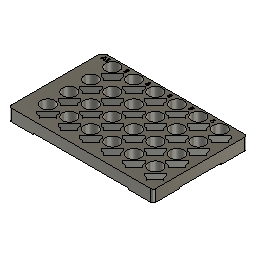
opentrons-tuberack-insert (Autodesk Fusion 360 design; units mm, degrees)
description: STEP AP214
part number: OpenTrons_1.5mL_rack
Autodesk Fusion 360 part; units mm, degrees
note: some values were not read from the file. Chosen so that the rebuilt part matches the saved one: which face or edge a step refers to.
(part 1 of 2)
imported_body "Base Feature1" makes body 1
other "Base Mesh Feature1"
sketch "Sketch1" plane through (0, 0, 0) normal (0, 0, 1) x (1, 0, 0)
  line L0 (-117.6969, -5.1718) -> (-116.414, -1.9968)
  line L1 (-116.414, -1.9968) -> (-115.8855, -1.9968)
  line L2 (-115.8855, -1.9968) -> (-114.6033, -5.1718)
  line L3 (-114.6033, -5.1718) -> (-115.2119, -5.1718)
  line L4 (-115.2119, -5.1718) -> (-115.4587, -4.5205)
  line L5 (-115.4587, -4.5205) -> (-116.8421, -4.5205)
  line L6 (-116.8421, -4.5205) -> (-117.0888, -5.1718)
  line L7 (-117.0888, -5.1718) -> (-117.6969, -5.1718)
  spline S0 degree 3 poles (-97.512, -2.4852) (-97.5271, -2.4858) (-97.5568, -2.4868) (-97.6004, -2.4938) (-97.6419, -2.5061) (-97.6818, -2.5226) (-97.7196, -2.5445) (-97.7552, -2.5715) (-97.789, -2.6028) (-97.8209, -2.6385) (-97.8499, -2.6783) (-97.8756, -2.7219) (-97.8969, -2.7692) (-97.9157, -2.8197) (-97.9302, -2.8738) (-97.9407, -2.9312) (-97.9487, -2.9919) (-97.9506, -3.0337) (-97.9515, -3.0551) knots 0 0 0 0 0.056467 0.111164 0.164937 0.218322 0.272393 0.327976 0.385291 0.444903 0.506844 0.569488 0.634153 0.700976 0.770897 0.843626 0.91966 1 1 1 1
  line L8 (-97.9515, -3.0551) -> (-98.5214, -3.0551)
  spline S1 degree 3 poles (-98.5214, -3.0551) (-98.5189, -3.012) (-98.5141, -2.9278) (-98.495, -2.8054) (-98.4693, -2.6898) (-98.4351, -2.5814) (-98.3922, -2.4801) (-98.3415, -2.3857) (-98.2819, -2.2986) (-98.2146, -2.2192) (-98.1407, -2.1481) (-98.0618, -2.085) (-97.9767, -2.0329) (-97.8869, -1.99) (-97.7924, -1.9558) (-97.6924, -1.9329) (-97.5878, -1.9174) (-97.5161, -1.9161) (-97.4796, -1.9154) knots 0 0 0 0 0.07494 0.146428 0.214753 0.280422 0.343604 0.405543 0.466199 0.526538 0.585902 0.64409 0.701613 0.758754 0.816629 0.875655 0.936624 1 1 1 1
  spline S2 degree 3 poles (-97.4796, -1.9154) (-97.4347, -1.9168) (-97.3472, -1.9195) (-97.22, -1.9428) (-97.1013, -1.9818) (-96.991, -2.0362) (-96.8902, -2.1054) (-96.7988, -2.1878) (-96.7196, -2.2854) (-96.6521, -2.3938) (-96.5961, -2.5087) (-96.5568, -2.6275) (-96.5309, -2.747) (-96.5282, -2.8275) (-96.5268, -2.8675) knots 0 0 0 0 0.089615 0.174949 0.257548 0.338901 0.420053 0.501401 0.584252 0.67037 0.756473 0.839207 0.92012 1 1 1 1
  spline S3 degree 3 poles (-96.5268, -2.8675) (-96.5274, -2.8917) (-96.5284, -2.9404) (-96.5359, -3.014) (-96.5471, -3.0891) (-96.5639, -3.1654) (-96.585, -3.2431) (-96.6105, -3.3223) (-96.6411, -3.4027) (-96.6762, -3.485) (-96.7181, -3.5697) (-96.767, -3.6579) (-96.824, -3.7495) (-96.8885, -3.8452) (-96.9608, -3.9447) (-97.0413, -4.0477) (-97.129, -4.1547) (-97.1913, -4.2262) (-97.2233, -4.2629) knots 0 0 0 0 0.045518 0.091616 0.139247 0.188242 0.238673 0.290664 0.34484 0.400432 0.459144 0.522551 0.590101 0.66226 0.739681 0.821575 0.90833 1 1 1 1
  line L9 (-97.2233, -4.2629) -> (-97.5546, -4.6426)
  line L10 (-97.5546, -4.6426) -> (-96.4861, -4.6426)
  line L11 (-96.4861, -4.6426) -> (-96.4861, -5.1718)
  line L12 (-96.4861, -5.1718) -> (-98.6028, -5.1718)
  line L13 (-98.6028, -5.1718) -> (-98.6028, -4.883)
  line L14 (-98.6028, -4.883) -> (-97.6628, -3.8826)
  spline S4 degree 3 poles (-97.6628, -3.8826) (-97.6355, -3.8534) (-97.5828, -3.7969) (-97.5078, -3.7139) (-97.44, -3.6351) (-97.3806, -3.5597) (-97.3267, -3.4902) (-97.2806, -3.4244) (-97.242, -3.363) (-97.2, -3.2889) (-97.1601, -3.2005) (-97.1236, -3.0987) (-97.1013, -3.0014) (-97.0982, -2.938) (-97.0967, -2.9076) knots 0 0 0 0 0.103844 0.201115 0.291116 0.374348 0.450707 0.52004 0.583258 0.639578 0.741537 0.83506 0.920873 1 1 1 1
  spline S5 degree 3 poles (-97.0967, -2.9076) (-97.0978, -2.8781) (-97.0999, -2.8211) (-97.1234, -2.74) (-97.1599, -2.6666) (-97.2112, -2.603) (-97.2734, -2.5508) (-97.3452, -2.5119) (-97.4261, -2.4895) (-97.4828, -2.4867) (-97.512, -2.4852) knots 0 0 0 0 0.132755 0.257234 0.378601 0.501406 0.623942 0.743642 0.868121 1 1 1 1
  line L15 (-62.7047, -3.9436) -> (-61.3856, -1.9154)
  line L16 (-61.3856, -1.9154) -> (-60.7916, -1.9154)
  line L17 (-60.7916, -1.9154) -> (-60.7916, -3.9913)
  line L18 (-60.7916, -3.9913) -> (-60.5066, -3.9913)
  line L19 (-60.5066, -3.9913) -> (-60.5066, -4.5205)
  line L20 (-60.5066, -4.5205) -> (-60.7916, -4.5205)
  line L21 (-60.7916, -4.5205) -> (-60.7916, -5.1718)
  line L22 (-60.7916, -5.1718) -> (-61.3614, -5.1718)
  line L23 (-61.3614, -5.1718) -> (-61.3614, -4.5205)
  line L24 (-61.3614, -4.5205) -> (-62.7047, -4.5205)
  line L25 (-62.7047, -4.5205) -> (-62.7047, -3.9436)
  line L26 (-25.9665, -3.5003) -> (-25.1601, -1.9154)
  line L27 (-25.1601, -1.9154) -> (-24.6557, -2.1711)
  line L28 (-24.6557, -2.1711) -> (-25.209, -3.2586)
  spline S6 degree 3 poles (-25.209, -3.2586) (-25.1763, -3.2595) (-25.112, -3.2612) (-25.0172, -3.2746) (-24.9266, -3.2979) (-24.8393, -3.3288) (-24.7563, -3.3703) (-24.6763, -3.4196) (-24.6014, -3.4797) (-24.5297, -3.5464) (-24.4646, -3.6202) (-24.408, -3.6996) (-24.3587, -3.7825) (-24.3204, -3.8708) (-24.2895, -3.9631) (-24.2672, -4.0598) (-24.2545, -4.161) (-24.2527, -4.2298) (-24.2518, -4.2648) knots 0 0 0 0 0.063329 0.124736 0.184916 0.2443 0.303826 0.364353 0.426073 0.489721 0.553756 0.616458 0.678319 0.740301 0.802656 0.866732 0.932157 1 1 1 1
  spline S7 degree 3 poles (-24.2518, -4.2648) (-24.2527, -4.2986) (-24.2543, -4.3653) (-24.268, -4.4633) (-24.2901, -4.5573) (-24.3217, -4.6471) (-24.3618, -4.7333) (-24.4109, -4.8156) (-24.4694, -4.8936) (-24.5357, -4.9668) (-24.6082, -5.0335) (-24.6846, -5.0927) (-24.7655, -5.1417) (-24.8495, -5.1831) (-24.9381, -5.2139) (-25.03, -5.2372) (-25.1257, -5.2506) (-25.1908, -5.2523) (-25.2237, -5.2532) knots 0 0 0 0 0.065621 0.129704 0.192008 0.253165 0.31459 0.376533 0.439287 0.503799 0.568284 0.630629 0.691513 0.751998 0.812377 0.873577 0.936027 1 1 1 1
  spline S8 degree 3 poles (-25.2237, -5.2532) (-25.2581, -5.2525) (-25.3257, -5.2511) (-25.4247, -5.2357) (-25.5197, -5.2124) (-25.61, -5.1792) (-25.6964, -5.1369) (-25.7776, -5.0845) (-25.8546, -5.0227) (-25.9264, -4.9529) (-25.991, -4.8763) (-26.0487, -4.7969) (-26.0975, -4.7143) (-26.137, -4.6289) (-26.1678, -4.5407) (-26.1892, -4.4496) (-26.2032, -4.356) (-26.2048, -4.2924) (-26.2057, -4.2604) knots 0 0 0 0 0.066486 0.130736 0.193287 0.255291 0.316538 0.378867 0.441877 0.507117 0.572271 0.635427 0.696817 0.757357 0.817265 0.877134 0.93802 1 1 1 1
  spline S9 degree 3 poles (-26.2057, -4.2604) (-26.2052, -4.2355) (-26.2044, -4.1857) (-26.1956, -4.1112) (-26.1822, -4.0364) (-26.1667, -3.9733) (-26.1507, -3.92) (-26.1346, -3.8748) (-26.1147, -3.8247) (-26.092, -3.7695) (-26.0656, -3.7093) (-26.0359, -3.6443) (-26.0026, -3.5739) (-25.9789, -3.5255) (-25.9665, -3.5003) knots 0 0 0 0 0.092538 0.185591 0.279552 0.375602 0.427617 0.487117 0.554199 0.628624 0.709688 0.799181 0.895357 1 1 1 1
  line L29 (-44.2093, -3.7586) -> (-43.836, -1.9968)
  line L30 (-43.836, -1.9968) -> (-42.3903, -1.9968)
  line L31 (-42.3903, -1.9968) -> (-42.3903, -2.5259)
  line L32 (-42.3903, -2.5259) -> (-43.3844, -2.5259)
  line L33 (-43.3844, -2.5259) -> (-43.5084, -3.1264)
  spline S10 degree 3 poles (-43.5084, -3.1264) (-43.4915, -3.1216) (-43.4582, -3.1124) (-43.408, -3.1031) (-43.3593, -3.097) (-43.3274, -3.0962) (-43.3119, -3.0958) knots 0 0 0 0 0.263654 0.51998 0.767103 1 1 1 1
  spline S11 degree 3 poles (-43.3119, -3.0958) (-43.2781, -3.0966) (-43.2116, -3.0981) (-43.1142, -3.1126) (-43.021, -3.1354) (-42.9322, -3.1679) (-42.8479, -3.2102) (-42.768, -3.2614) (-42.6924, -3.3216) (-42.6224, -3.3908) (-42.5582, -3.4667) (-42.5023, -3.5489) (-42.4546, -3.636) (-42.4166, -3.7288) (-42.3866, -3.8265) (-42.365, -3.9293) (-42.3522, -4.0372) (-42.3505, -4.1109) (-42.3496, -4.1484) knots 0 0 0 0 0.063401 0.124976 0.184492 0.243474 0.302264 0.361384 0.421482 0.483455 0.545936 0.608143 0.66982 0.732332 0.796092 0.861643 0.929435 1 1 1 1
  spline S12 degree 3 poles (-42.3496, -4.1484) (-42.3507, -4.1864) (-42.3528, -4.2614) (-42.3666, -4.3716) (-42.3911, -4.4771) (-42.4247, -4.5783) (-42.4689, -4.6744) (-42.5221, -4.7664) (-42.5852, -4.8535) (-42.6575, -4.935) (-42.7361, -5.0094) (-42.8199, -5.0749) (-42.9081, -5.13) (-43.0008, -5.1746) (-43.0975, -5.2098) (-43.1982, -5.2355) (-43.3034, -5.2502) (-43.3748, -5.2522) (-43.4111, -5.2532) knots 0 0 0 0 0.066755 0.131728 0.19481 0.256899 0.318751 0.380351 0.443324 0.507463 0.571506 0.633361 0.693942 0.753929 0.813802 0.874524 0.936222 1 1 1 1
  spline S13 degree 3 poles (-43.4111, -5.2532) (-43.4436, -5.2524) (-43.5076, -5.2507) (-43.6019, -5.2407) (-43.6928, -5.2229) (-43.7798, -5.1972) (-43.8639, -5.1655) (-43.9441, -5.1259) (-44.0208, -5.0791) (-44.0938, -5.0259) (-44.1619, -4.9661) (-44.224, -4.9006) (-44.2806, -4.8302) (-44.3304, -4.7542) (-44.3733, -4.6725) (-44.4113, -4.5862) (-44.4424, -4.4944) (-44.4582, -4.4307) (-44.4663, -4.3984) knots 0 0 0 0 0.065935 0.130037 0.192362 0.25382 0.314199 0.37467 0.435154 0.496479 0.557809 0.619031 0.679691 0.740961 0.803375 0.866818 0.932318 1 1 1 1
  line L34 (-44.4663, -4.3984) -> (-43.815, -4.3984)
  spline S14 degree 3 poles (-43.815, -4.3984) (-43.8031, -4.4208) (-43.7799, -4.4644) (-43.7359, -4.5222) (-43.6866, -4.5715) (-43.6326, -4.6128) (-43.5733, -4.6438) (-43.5113, -4.6672) (-43.4458, -4.6808) (-43.4012, -4.6825) (-43.3787, -4.6833) knots 0 0 0 0 0.138114 0.268408 0.394191 0.517092 0.637493 0.757004 0.877294 1 1 1 1
  spline S15 degree 3 poles (-43.3787, -4.6833) (-43.363, -4.6827) (-43.3321, -4.6816) (-43.2865, -4.6754) (-43.2431, -4.6638) (-43.2014, -4.6476) (-43.1613, -4.6275) (-43.1234, -4.6021) (-43.0871, -4.5729) (-43.0529, -4.5394) (-43.0219, -4.502) (-42.9947, -4.4618) (-42.9704, -4.4197) (-42.9524, -4.3741) (-42.9377, -4.3262) (-42.9268, -4.2758) (-42.9204, -4.2228) (-42.9198, -4.1866) (-42.9195, -4.1681) knots 0 0 0 0 0.061179 0.120371 0.178442 0.235934 0.294268 0.352654 0.413122 0.475586 0.5389 0.601869 0.664333 0.727647 0.792409 0.85912 0.928135 1 1 1 1
  spline S16 degree 3 poles (-42.9195, -4.1681) (-42.9198, -4.1501) (-42.9205, -4.115) (-42.9262, -4.0635) (-42.9365, -4.0146) (-42.9504, -3.9679) (-42.9683, -3.9238) (-42.9901, -3.882) (-43.016, -3.8427) (-43.0461, -3.8067) (-43.0782, -3.7736) (-43.1126, -3.7447) (-43.1492, -3.7207) (-43.1867, -3.6998) (-43.2266, -3.6846) (-43.268, -3.6741) (-43.311, -3.6664) (-43.3403, -3.6659) (-43.3551, -3.6657) knots 0 0 0 0 0.072891 0.141883 0.209282 0.274623 0.338439 0.401305 0.465006 0.52832 0.59074 0.650981 0.70969 0.767212 0.824188 0.881767 0.939955 1 1 1 1
  spline S17 degree 3 poles (-43.3551, -3.6657) (-43.3713, -3.6663) (-43.4037, -3.6675) (-43.4518, -3.6775) (-43.4993, -3.6937) (-43.5465, -3.716) (-43.593, -3.7453) (-43.6399, -3.7795) (-43.6856, -3.8213) (-43.7147, -3.8525) (-43.7297, -3.8686) knots 0 0 0 0 0.11036 0.221186 0.334364 0.452977 0.577234 0.708804 0.849355 1 1 1 1
  line L35 (-43.7297, -3.8686) -> (-44.2093, -3.7586)
  spline S18 degree 3 poles (-79.3483, -2.4852) (-79.369, -2.4863) (-79.41, -2.4883) (-79.4699, -2.5033) (-79.5268, -2.5287) (-79.5795, -2.5636) (-79.6272, -2.6056) (-79.6664, -2.6553) (-79.699, -2.7097) (-79.7128, -2.7499) (-79.7198, -2.7702) knots 0 0 0 0 0.123523 0.245107 0.367266 0.494691 0.622324 0.746003 0.872253 1 1 1 1
  line L36 (-79.7198, -2.7702) -> (-80.2896, -2.7702)
  spline S19 degree 3 poles (-80.2896, -2.7702) (-80.2856, -2.7417) (-80.2777, -2.6859) (-80.2589, -2.605) (-80.2363, -2.5283) (-80.2081, -2.456) (-80.175, -2.388) (-80.1375, -2.324) (-80.0949, -2.2644) (-80.0623, -2.2284) (-80.0461, -2.2105) knots 0 0 0 0 0.138934 0.272371 0.400702 0.524915 0.646775 0.765706 0.883115 1 1 1 1
  spline S20 degree 3 poles (-80.0461, -2.2105) (-80.0226, -2.1868) (-79.9764, -2.1402) (-79.8991, -2.0805) (-79.8181, -2.0288) (-79.7318, -1.9878) (-79.6414, -1.9546) (-79.5464, -1.9324) (-79.447, -1.9176) (-79.3791, -1.9161) (-79.3445, -1.9154) knots 0 0 0 0 0.127407 0.251106 0.372908 0.494496 0.616171 0.740563 0.867605 1 1 1 1
  spline S21 degree 3 poles (-79.3445, -1.9154) (-79.3138, -1.9161) (-79.2533, -1.9175) (-79.1644, -1.929) (-79.0796, -1.9491) (-78.9981, -1.9754) (-78.921, -2.0112) (-78.8467, -2.0527) (-78.7771, -2.1036) (-78.7123, -2.1612) (-78.6527, -2.2234) (-78.6011, -2.2899) (-78.5567, -2.359) (-78.5202, -2.4311) (-78.4921, -2.5064) (-78.4726, -2.5845) (-78.4598, -2.6652) (-78.4586, -2.7201) (-78.4579, -2.7479) knots 0 0 0 0 0.068214 0.134095 0.198286 0.26116 0.323635 0.386367 0.449642 0.514245 0.578413 0.640375 0.700615 0.760104 0.819299 0.878466 0.93836 1 1 1 1
  spline S22 degree 3 poles (-78.4579, -2.7479) (-78.4592, -2.7824) (-78.4618, -2.8502) (-78.4832, -2.9495) (-78.5167, -3.0444) (-78.565, -3.1337) (-78.6255, -3.217) (-78.6996, -3.2916) (-78.7854, -3.3587) (-78.8498, -3.3947) (-78.8828, -3.4132) knots 0 0 0 0 0.124101 0.244316 0.364466 0.485854 0.608915 0.734301 0.863943 1 1 1 1
  spline S23 degree 3 poles (-78.8828, -3.4132) (-78.8601, -3.4206) (-78.8157, -3.4352) (-78.7525, -3.464) (-78.6924, -3.4954) (-78.6364, -3.5319) (-78.584, -3.572) (-78.5355, -3.6161) (-78.4907, -3.664) (-78.4502, -3.716) (-78.4142, -3.7714) (-78.3819, -3.8287) (-78.3554, -3.8889) (-78.3329, -3.9513) (-78.3157, -4.0164) (-78.3037, -4.084) (-78.2967, -4.154) (-78.2956, -4.2014) (-78.2951, -4.2254) knots 0 0 0 0 0.066221 0.130122 0.192922 0.254764 0.315757 0.376303 0.436814 0.498168 0.559516 0.620243 0.68097 0.742349 0.804584 0.868102 0.933307 1 1 1 1
  spline S24 degree 3 poles (-78.2951, -4.2254) (-78.2962, -4.2606) (-78.2983, -4.3301) (-78.312, -4.4324) (-78.3374, -4.5299) (-78.3709, -4.6238) (-78.4155, -4.7129) (-78.4681, -4.7991) (-78.5326, -4.8796) (-78.6044, -4.9563) (-78.6841, -5.0261) (-78.7705, -5.0866) (-78.8617, -5.1385) (-78.9583, -5.1806) (-79.0602, -5.2131) (-79.1673, -5.2366) (-79.2799, -5.2509) (-79.3568, -5.2524) (-79.396, -5.2532) knots 0 0 0 0 0.062821 0.123871 0.183554 0.242266 0.301265 0.360847 0.421949 0.484789 0.548014 0.610413 0.672536 0.734829 0.797947 0.862973 0.93002 1 1 1 1
  spline S25 degree 3 poles (-79.396, -5.2532) (-79.4332, -5.2524) (-79.5058, -5.2508) (-79.6121, -5.2371) (-79.713, -5.215) (-79.809, -5.1838) (-79.8995, -5.1433) (-79.9856, -5.0952) (-80.0653, -5.0366) (-80.1396, -4.9701) (-80.2069, -4.8955) (-80.2671, -4.8145) (-80.3188, -4.7268) (-80.3622, -4.6329) (-80.397, -4.5324) (-80.4245, -4.4257) (-80.4436, -4.3125) (-80.4495, -4.2346) (-80.4525, -4.1949) knots 0 0 0 0 0.066659 0.130343 0.191936 0.251996 0.311122 0.369755 0.428602 0.488436 0.548524 0.608661 0.669236 0.730881 0.794196 0.85983 0.928533 1 1 1 1
  line L37 (-80.4525, -4.1949) -> (-79.8826, -4.1949)
  spline S26 degree 3 poles (-79.8826, -4.1949) (-79.879, -4.2148) (-79.872, -4.2537) (-79.8582, -4.31) (-79.8404, -4.362) (-79.8197, -4.4101) (-79.7974, -4.455) (-79.7704, -4.495) (-79.7407, -4.5311) (-79.6979, -4.5741) (-79.6368, -4.6183) (-79.5542, -4.6567) (-79.4623, -4.6792) (-79.3981, -4.6819) (-79.3649, -4.6833) knots 0 0 0 0 0.077346 0.150652 0.220677 0.286575 0.350188 0.411379 0.469946 0.528234 0.642194 0.755364 0.873556 1 1 1 1
  spline S27 degree 3 poles (-79.3649, -4.6833) (-79.3473, -4.683) (-79.3128, -4.6824) (-79.2621, -4.6759) (-79.2138, -4.6651) (-79.1678, -4.6504) (-79.1239, -4.632) (-79.0828, -4.6083) (-79.0437, -4.5807) (-79.007, -4.5497) (-78.9732, -4.5159) (-78.945, -4.4784) (-78.9193, -4.4404) (-78.9002, -4.3993) (-78.8836, -4.3573) (-78.8734, -4.3129) (-78.8656, -4.267) (-78.8652, -4.2356) (-78.865, -4.2197) knots 0 0 0 0 0.069402 0.135943 0.20102 0.264181 0.325955 0.388454 0.450819 0.514266 0.577492 0.638835 0.698634 0.758057 0.817032 0.876415 0.937278 1 1 1 1
  spline S28 degree 3 poles (-78.865, -4.2197) (-78.8656, -4.2022) (-78.8668, -4.1675) (-78.8766, -4.1169) (-78.8921, -4.0682) (-78.9136, -4.0216) (-78.9424, -3.9774) (-78.9763, -3.9346) (-79.0181, -3.8954) (-79.064, -3.8567) (-79.1172, -3.823) (-79.1751, -3.7918) (-79.2392, -3.7671) (-79.308, -3.7449) (-79.3829, -3.7288) (-79.4632, -3.717) (-79.5489, -3.7083) (-79.608, -3.707) (-79.6384, -3.7064) knots 0 0 0 0 0.050613 0.10076 0.149275 0.198888 0.249306 0.302323 0.357221 0.415437 0.476443 0.539829 0.606184 0.675941 0.749782 0.828288 0.911845 1 1 1 1
  line L38 (-79.6384, -3.7064) -> (-79.6384, -3.1772)
  spline S29 degree 3 poles (-79.6384, -3.1772) (-79.6006, -3.174) (-79.5299, -3.168) (-79.4318, -3.1539) (-79.3492, -3.1351) (-79.2802, -3.1124) (-79.2229, -3.0833) (-79.1728, -3.0511) (-79.1296, -3.0137) (-79.0932, -2.9723) (-79.064, -2.9278) (-79.0434, -2.8809) (-79.0297, -2.8331) (-79.0284, -2.8004) (-79.0278, -2.7842) knots 0 0 0 0 0.141704 0.2651 0.370058 0.458024 0.535994 0.609848 0.680075 0.748587 0.81563 0.878071 0.939584 1 1 1 1
  spline S30 degree 3 poles (-79.0278, -2.7842) (-79.0289, -2.7635) (-79.031, -2.7232) (-79.0478, -2.6654) (-79.0768, -2.6139) (-79.1158, -2.5688) (-79.1633, -2.5312) (-79.2189, -2.5038) (-79.2815, -2.4878) (-79.3256, -2.4861) (-79.3483, -2.4852) knots 0 0 0 0 0.126208 0.246331 0.363484 0.484754 0.608383 0.731214 0.860989 1 1 1 1
  line L39 (-114.1352, -2.5259) -> (-113.7949, -1.9968)
  line L40 (-113.7949, -1.9968) -> (-112.914, -1.9968)
  line L41 (-112.914, -1.9968) -> (-112.914, -5.1718)
  line L42 (-112.914, -5.1718) -> (-113.4839, -5.1718)
  line L43 (-113.4839, -5.1718) -> (-113.4839, -2.5259)
  line L44 (-113.4839, -2.5259) -> (-114.1352, -2.5259)
  line L45 (-2, 0) -> (-117, 0)
  line L46 (-121, -4) -> (-121, -76.75)
  line L47 (-119, -78.75) -> (-2, -78.75)
  line L48 (0, -76.75) -> (0, -2)
  line L49 (-16.0663, -16.324) -> (-6.591, -6.8487)
  line L50 (-4.8233, -8.6165) -> (-6.591, -6.8487)
  line L51 (-4.8233, -8.6165) -> (-4.2576, -11.5864)
  line L52 (-4.2576, -11.5864) -> (-11.3286, -18.6574)
  line L53 (-11.3286, -18.6574) -> (-14.2985, -18.0917)
  line L54 (-14.2985, -18.0917) -> (-16.0663, -16.324)
  line L55 (-11.3286, -11.5864) -> (-16.19, -6.725) construction
  line L56 (-121, -4) -> (-117, 0)
  circle A0 centre (-16.19, -6.725) radius 5.675
  arc A1 (0, -2) -> (-2, 0) centre (-2, -2) ccw
  arc A2 (-2, -78.75) -> (0, -76.75) centre (-2, -76.75) ccw
  arc A3 (-121, -76.75) -> (-119, -78.75) centre (-119, -76.75) ccw
  line L57 (-100.5, -78.75) -> (-100.5, -76.75)
  line L58 (-20.5, -76.75) -> (-20.5, -78.75)
  line L59 (-20.5, -76.75) -> (-100.5, -76.75)
  line L60 (0, -39.375) -> (-121, -39.375) construction
  line L61 (-20.5, -2) -> (-100.5, -2)
  line L62 (-100.5, 0) -> (-100.5, -2)
  line L63 (-20.5, -2) -> (-20.5, 0)
  line L64 (-11.3286, -18.6574) -> (-9.9144, -20.0716)
  line L65 (-9.9144, -20.0716) -> (-2.8434, -13.0006)
  line L66 (-2.8434, -13.0006) -> (-4.2576, -11.5864)
  line L67 (-16.19, -6.725) -> (0, -6.725) construction
  line L68 (-98.5214, -3.0551) -> (-98.5189, -3.012) construction
  line L69 (-98.5189, -3.012) -> (-98.5141, -2.9278) construction
  line L70 (-98.5141, -2.9278) -> (-98.495, -2.8054) construction
  line L71 (-98.495, -2.8054) -> (-98.4693, -2.6898) construction
  line L72 (-98.4693, -2.6898) -> (-98.4351, -2.5814) construction
  line L73 (-98.4351, -2.5814) -> (-98.3922, -2.4801) construction
  line L74 (-98.3922, -2.4801) -> (-98.3415, -2.3857) construction
  line L75 (-98.3415, -2.3857) -> (-98.2819, -2.2986) construction
  line L76 (-98.2819, -2.2986) -> (-98.2146, -2.2192) construction
  line L77 (-98.2146, -2.2192) -> (-98.1407, -2.1481) construction
  line L78 (-98.1407, -2.1481) -> (-98.0618, -2.085) construction
  line L79 (-98.0618, -2.085) -> (-97.9767, -2.0329) construction
  line L80 (-97.9767, -2.0329) -> (-97.8869, -1.99) construction
  line L81 (-97.8869, -1.99) -> (-97.7924, -1.9558) construction
  line L82 (-97.7924, -1.9558) -> (-97.6924, -1.9329) construction
  line L83 (-97.6924, -1.9329) -> (-97.5878, -1.9174) construction
  line L84 (-97.5878, -1.9174) -> (-97.5161, -1.9161) construction
  line L85 (-97.5161, -1.9161) -> (-97.4796, -1.9154) construction
  line L86 (-97.4796, -1.9154) -> (-97.4347, -1.9168) construction
  line L87 (-97.4347, -1.9168) -> (-97.3472, -1.9195) construction
  line L88 (-97.3472, -1.9195) -> (-97.22, -1.9428) construction
  line L89 (-97.22, -1.9428) -> (-97.1013, -1.9818) construction
  line L90 (-97.1013, -1.9818) -> (-96.991, -2.0362) construction
  line L91 (-96.991, -2.0362) -> (-96.8902, -2.1054) construction
  line L92 (-96.8902, -2.1054) -> (-96.7988, -2.1878) construction
  line L93 (-96.7988, -2.1878) -> (-96.7196, -2.2854) construction
  line L94 (-96.7196, -2.2854) -> (-96.6521, -2.3938) construction
  line L95 (-96.6521, -2.3938) -> (-96.5961, -2.5087) construction
  line L96 (-96.5961, -2.5087) -> (-96.5568, -2.6275) construction
  line L97 (-96.5568, -2.6275) -> (-96.5309, -2.747) construction
  line L98 (-96.5309, -2.747) -> (-96.5282, -2.8275) construction
  line L99 (-96.5282, -2.8275) -> (-96.5268, -2.8675) construction
  line L100 (-97.6628, -3.8826) -> (-97.6355, -3.8534) construction
  line L101 (-97.6355, -3.8534) -> (-97.5828, -3.7969) construction
  line L102 (-97.5828, -3.7969) -> (-97.5078, -3.7139) construction
  line L103 (-97.5078, -3.7139) -> (-97.44, -3.6351) construction
  line L104 (-97.44, -3.6351) -> (-97.3806, -3.5597) construction
  line L105 (-97.3806, -3.5597) -> (-97.3267, -3.4902) construction
  line L106 (-97.3267, -3.4902) -> (-97.2806, -3.4244) construction
  line L107 (-97.2806, -3.4244) -> (-97.242, -3.363) construction
  line L108 (-97.242, -3.363) -> (-97.2, -3.2889) construction
  line L109 (-97.2, -3.2889) -> (-97.1601, -3.2005) construction
  line L110 (-97.1601, -3.2005) -> (-97.1236, -3.0987) construction
  line L111 (-97.1236, -3.0987) -> (-97.1013, -3.0014) construction
  line L112 (-97.1013, -3.0014) -> (-97.0982, -2.938) construction
  line L113 (-97.0982, -2.938) -> (-97.0967, -2.9076) construction
  line L114 (-97.512, -2.4852) -> (-97.5271, -2.4858) construction
  line L115 (-97.5271, -2.4858) -> (-97.5568, -2.4868) construction
  line L116 (-97.5568, -2.4868) -> (-97.6004, -2.4938) construction
  line L117 (-97.6004, -2.4938) -> (-97.6419, -2.5061) construction
  line L118 (-97.6419, -2.5061) -> (-97.6818, -2.5226) construction
  line L119 (-97.6818, -2.5226) -> (-97.7196, -2.5445) construction
  line L120 (-97.7196, -2.5445) -> (-97.7552, -2.5715) construction
  line L121 (-97.7552, -2.5715) -> (-97.789, -2.6028) construction
  line L122 (-97.789, -2.6028) -> (-97.8209, -2.6385) construction
  line L123 (-97.8209, -2.6385) -> (-97.8499, -2.6783) construction
  line L124 (-97.8499, -2.6783) -> (-97.8756, -2.7219) construction
  line L125 (-97.8756, -2.7219) -> (-97.8969, -2.7692) construction
  line L126 (-97.8969, -2.7692) -> (-97.9157, -2.8197) construction
  line L127 (-97.9157, -2.8197) -> (-97.9302, -2.8738) construction
  line L128 (-97.9302, -2.8738) -> (-97.9407, -2.9312) construction
  line L129 (-97.9407, -2.9312) -> (-97.9487, -2.9919) construction
  line L130 (-97.9487, -2.9919) -> (-97.9506, -3.0337) construction
  line L131 (-97.9506, -3.0337) -> (-97.9515, -3.0551) construction
  line L132 (-97.0967, -2.9076) -> (-97.0978, -2.8781) construction
  line L133 (-97.0978, -2.8781) -> (-97.0999, -2.8211) construction
  line L134 (-97.0999, -2.8211) -> (-97.1234, -2.74) construction
  line L135 (-97.1234, -2.74) -> (-97.1599, -2.6666) construction
  line L136 (-97.1599, -2.6666) -> (-97.2112, -2.603) construction
  line L137 (-97.2112, -2.603) -> (-97.2734, -2.5508) construction
  line L138 (-97.2734, -2.5508) -> (-97.3452, -2.5119) construction
  line L139 (-97.3452, -2.5119) -> (-97.4261, -2.4895) construction
  line L140 (-97.4261, -2.4895) -> (-97.4828, -2.4867) construction
  line L141 (-97.4828, -2.4867) -> (-97.512, -2.4852) construction
  line L142 (-96.5268, -2.8675) -> (-96.5274, -2.8917) construction
  line L143 (-96.5274, -2.8917) -> (-96.5284, -2.9404) construction
  line L144 (-96.5284, -2.9404) -> (-96.5359, -3.014) construction
  line L145 (-96.5359, -3.014) -> (-96.5471, -3.0891) construction
  line L146 (-96.5471, -3.0891) -> (-96.5639, -3.1654) construction
  line L147 (-96.5639, -3.1654) -> (-96.585, -3.2431) construction
  line L148 (-96.585, -3.2431) -> (-96.6105, -3.3223) construction
  line L149 (-96.6105, -3.3223) -> (-96.6411, -3.4027) construction
  line L150 (-96.6411, -3.4027) -> (-96.6762, -3.485) construction
  line L151 (-96.6762, -3.485) -> (-96.7181, -3.5697) construction
  line L152 (-96.7181, -3.5697) -> (-96.767, -3.6579) construction
  line L153 (-96.767, -3.6579) -> (-96.824, -3.7495) construction
  line L154 (-96.824, -3.7495) -> (-96.8885, -3.8452) construction
  line L155 (-96.8885, -3.8452) -> (-96.9608, -3.9447) construction
  line L156 (-96.9608, -3.9447) -> (-97.0413, -4.0477) construction
  line L157 (-97.0413, -4.0477) -> (-97.129, -4.1547) construction
  line L158 (-97.129, -4.1547) -> (-97.1913, -4.2262) construction
  line L159 (-97.1913, -4.2262) -> (-97.2233, -4.2629) construction
  line L160 (-79.396, -5.2532) -> (-79.4332, -5.2524) construction
  line L161 (-79.4332, -5.2524) -> (-79.5058, -5.2508) construction
  line L162 (-79.5058, -5.2508) -> (-79.6121, -5.2371) construction
  line L163 (-79.6121, -5.2371) -> (-79.713, -5.215) construction
  line L164 (-79.713, -5.215) -> (-79.809, -5.1838) construction
  line L165 (-79.809, -5.1838) -> (-79.8995, -5.1433) construction
  line L166 (-79.8995, -5.1433) -> (-79.9856, -5.0952) construction
  line L167 (-79.9856, -5.0952) -> (-80.0653, -5.0366) construction
  line L168 (-80.0653, -5.0366) -> (-80.1396, -4.9701) construction
  line L169 (-80.1396, -4.9701) -> (-80.2069, -4.8955) construction
  line L170 (-80.2069, -4.8955) -> (-80.2671, -4.8145) construction
  line L171 (-80.2671, -4.8145) -> (-80.3188, -4.7268) construction
  line L172 (-80.3188, -4.7268) -> (-80.3622, -4.6329) construction
  line L173 (-80.3622, -4.6329) -> (-80.397, -4.5324) construction
  line L174 (-80.397, -4.5324) -> (-80.4245, -4.4257) construction
  line L175 (-80.4245, -4.4257) -> (-80.4436, -4.3125) construction
  line L176 (-80.4436, -4.3125) -> (-80.4495, -4.2346) construction
  line L177 (-80.4495, -4.2346) -> (-80.4525, -4.1949) construction
  line L178 (-79.8826, -4.1949) -> (-79.879, -4.2148) construction
  line L179 (-79.879, -4.2148) -> (-79.872, -4.2537) construction
  line L180 (-79.872, -4.2537) -> (-79.8582, -4.31) construction
  line L181 (-79.8582, -4.31) -> (-79.8404, -4.362) construction
  line L182 (-79.8404, -4.362) -> (-79.8197, -4.4101) construction
  line L183 (-79.8197, -4.4101) -> (-79.7974, -4.455) construction
  line L184 (-79.7974, -4.455) -> (-79.7704, -4.495) construction
  line L185 (-79.7704, -4.495) -> (-79.7407, -4.5311) construction
  line L186 (-79.7407, -4.5311) -> (-79.6979, -4.5741) construction
  line L187 (-79.6979, -4.5741) -> (-79.6368, -4.6183) construction
  line L188 (-79.6368, -4.6183) -> (-79.5542, -4.6567) construction
  line L189 (-79.5542, -4.6567) -> (-79.4623, -4.6792) construction
  line L190 (-79.4623, -4.6792) -> (-79.3981, -4.6819) construction
  line L191 (-79.3981, -4.6819) -> (-79.3649, -4.6833) construction
  line L192 (-79.3649, -4.6833) -> (-79.3473, -4.683) construction
  line L193 (-79.3473, -4.683) -> (-79.3128, -4.6824) construction
  line L194 (-79.3128, -4.6824) -> (-79.2621, -4.6759) construction
  line L195 (-79.2621, -4.6759) -> (-79.2138, -4.6651) construction
  line L196 (-79.2138, -4.6651) -> (-79.1678, -4.6504) construction
  line L197 (-79.1678, -4.6504) -> (-79.1239, -4.632) construction
  line L198 (-79.1239, -4.632) -> (-79.0828, -4.6083) construction
  line L199 (-79.0828, -4.6083) -> (-79.0437, -4.5807) construction
  line L200 (-79.0437, -4.5807) -> (-79.007, -4.5497) construction
  line L201 (-79.007, -4.5497) -> (-78.9732, -4.5159) construction
  line L202 (-78.9732, -4.5159) -> (-78.945, -4.4784) construction
  line L203 (-78.945, -4.4784) -> (-78.9193, -4.4404) construction
  line L204 (-78.9193, -4.4404) -> (-78.9002, -4.3993) construction
  line L205 (-78.9002, -4.3993) -> (-78.8836, -4.3573) construction
  line L206 (-78.8836, -4.3573) -> (-78.8734, -4.3129) construction
  line L207 (-78.8734, -4.3129) -> (-78.8656, -4.267) construction
  line L208 (-78.8656, -4.267) -> (-78.8652, -4.2356) construction
  line L209 (-78.8652, -4.2356) -> (-78.865, -4.2197) construction
  line L210 (-78.865, -4.2197) -> (-78.8656, -4.2022) construction
  line L211 (-78.8656, -4.2022) -> (-78.8668, -4.1675) construction
  line L212 (-78.8668, -4.1675) -> (-78.8766, -4.1169) construction
  line L213 (-78.8766, -4.1169) -> (-78.8921, -4.0682) construction
  line L214 (-78.8921, -4.0682) -> (-78.9136, -4.0216) construction
  line L215 (-78.9136, -4.0216) -> (-78.9424, -3.9774) construction
  line L216 (-78.9424, -3.9774) -> (-78.9763, -3.9346) construction
  line L217 (-78.9763, -3.9346) -> (-79.0181, -3.8954) construction
  line L218 (-79.0181, -3.8954) -> (-79.064, -3.8567) construction
  line L219 (-79.064, -3.8567) -> (-79.1172, -3.823) construction
  line L220 (-79.1172, -3.823) -> (-79.1751, -3.7918) construction
  line L221 (-79.1751, -3.7918) -> (-79.2392, -3.7671) construction
  line L222 (-79.2392, -3.7671) -> (-79.308, -3.7449) construction
  line L223 (-79.308, -3.7449) -> (-79.3829, -3.7288) construction
  line L224 (-79.3829, -3.7288) -> (-79.4632, -3.717) construction
  line L225 (-79.4632, -3.717) -> (-79.5489, -3.7083) construction
  line L226 (-79.5489, -3.7083) -> (-79.608, -3.707) construction
  line L227 (-79.608, -3.707) -> (-79.6384, -3.7064) construction
  line L228 (-79.6384, -3.1772) -> (-79.6006, -3.174) construction
  line L229 (-79.6006, -3.174) -> (-79.5299, -3.168) construction
  line L230 (-79.5299, -3.168) -> (-79.4318, -3.1539) construction
  line L231 (-79.4318, -3.1539) -> (-79.3492, -3.1351) construction
  line L232 (-79.3492, -3.1351) -> (-79.2802, -3.1124) construction
  line L233 (-79.2802, -3.1124) -> (-79.2229, -3.0833) construction
  line L234 (-79.2229, -3.0833) -> (-79.1728, -3.0511) construction
  line L235 (-79.1728, -3.0511) -> (-79.1296, -3.0137) construction
  line L236 (-79.1296, -3.0137) -> (-79.0932, -2.9723) construction
  line L237 (-79.0932, -2.9723) -> (-79.064, -2.9278) construction
  line L238 (-79.064, -2.9278) -> (-79.0434, -2.8809) construction
  line L239 (-79.0434, -2.8809) -> (-79.0297, -2.8331) construction
  line L240 (-79.0297, -2.8331) -> (-79.0284, -2.8004) construction
  line L241 (-79.0284, -2.8004) -> (-79.0278, -2.7842) construction
  line L242 (-79.0278, -2.7842) -> (-79.0289, -2.7635) construction
  line L243 (-79.0289, -2.7635) -> (-79.031, -2.7232) construction
  line L244 (-79.031, -2.7232) -> (-79.0478, -2.6654) construction
  line L245 (-79.0478, -2.6654) -> (-79.0768, -2.6139) construction
  line L246 (-79.0768, -2.6139) -> (-79.1158, -2.5688) construction
  line L247 (-79.1158, -2.5688) -> (-79.1633, -2.5312) construction
  line L248 (-79.1633, -2.5312) -> (-79.2189, -2.5038) construction
  line L249 (-79.2189, -2.5038) -> (-79.2815, -2.4878) construction
  line L250 (-79.2815, -2.4878) -> (-79.3256, -2.4861) construction
  line L251 (-79.3256, -2.4861) -> (-79.3483, -2.4852) construction
  line L252 (-79.3483, -2.4852) -> (-79.369, -2.4863) construction
  line L253 (-79.369, -2.4863) -> (-79.41, -2.4883) construction
  line L254 (-79.41, -2.4883) -> (-79.4699, -2.5033) construction
  line L255 (-79.4699, -2.5033) -> (-79.5268, -2.5287) construction
  line L256 (-79.5268, -2.5287) -> (-79.5795, -2.5636) construction
  line L257 (-79.5795, -2.5636) -> (-79.6272, -2.6056) construction
  line L258 (-79.6272, -2.6056) -> (-79.6664, -2.6553) construction
  line L259 (-79.6664, -2.6553) -> (-79.699, -2.7097) construction
  line L260 (-79.699, -2.7097) -> (-79.7128, -2.7499) construction
  line L261 (-79.7128, -2.7499) -> (-79.7198, -2.7702) construction
  line L262 (-80.2896, -2.7702) -> (-80.2856, -2.7417) construction
  line L263 (-80.2856, -2.7417) -> (-80.2777, -2.6859) construction
  line L264 (-80.2777, -2.6859) -> (-80.2589, -2.605) construction
  line L265 (-80.2589, -2.605) -> (-80.2363, -2.5283) construction
  line L266 (-80.2363, -2.5283) -> (-80.2081, -2.456) construction
  line L267 (-80.2081, -2.456) -> (-80.175, -2.388) construction
  line L268 (-80.175, -2.388) -> (-80.1375, -2.324) construction
  line L269 (-80.1375, -2.324) -> (-80.0949, -2.2644) construction
  line L270 (-80.0949, -2.2644) -> (-80.0623, -2.2284) construction
  line L271 (-80.0623, -2.2284) -> (-80.0461, -2.2105) construction
  line L272 (-80.0461, -2.2105) -> (-80.0226, -2.1868) construction
  line L273 (-80.0226, -2.1868) -> (-79.9764, -2.1402) construction
  line L274 (-79.9764, -2.1402) -> (-79.8991, -2.0805) construction
  line L275 (-79.8991, -2.0805) -> (-79.8181, -2.0288) construction
  line L276 (-79.8181, -2.0288) -> (-79.7318, -1.9878) construction
  line L277 (-79.7318, -1.9878) -> (-79.6414, -1.9546) construction
  line L278 (-79.6414, -1.9546) -> (-79.5464, -1.9324) construction
  line L279 (-79.5464, -1.9324) -> (-79.447, -1.9176) construction
  line L280 (-79.447, -1.9176) -> (-79.3791, -1.9161) construction
  line L281 (-79.3791, -1.9161) -> (-79.3445, -1.9154) construction
  line L282 (-79.3445, -1.9154) -> (-79.3138, -1.9161) construction
  line L283 (-79.3138, -1.9161) -> (-79.2533, -1.9175) construction
  line L284 (-79.2533, -1.9175) -> (-79.1644, -1.929) construction
  line L285 (-79.1644, -1.929) -> (-79.0796, -1.9491) construction
  line L286 (-79.0796, -1.9491) -> (-78.9981, -1.9754) construction
  line L287 (-78.9981, -1.9754) -> (-78.921, -2.0112) construction
  line L288 (-78.921, -2.0112) -> (-78.8467, -2.0527) construction
  line L289 (-78.8467, -2.0527) -> (-78.7771, -2.1036) construction
  line L290 (-78.7771, -2.1036) -> (-78.7123, -2.1612) construction
  line L291 (-78.7123, -2.1612) -> (-78.6527, -2.2234) construction
  line L292 (-78.6527, -2.2234) -> (-78.6011, -2.2899) construction
  line L293 (-78.6011, -2.2899) -> (-78.5567, -2.359) construction
  line L294 (-78.5567, -2.359) -> (-78.5202, -2.4311) construction
  line L295 (-78.5202, -2.4311) -> (-78.4921, -2.5064) construction
  line L296 (-78.4921, -2.5064) -> (-78.4726, -2.5845) construction
  line L297 (-78.4726, -2.5845) -> (-78.4598, -2.6652) construction
  line L298 (-78.4598, -2.6652) -> (-78.4586, -2.7201) construction
  line L299 (-78.4586, -2.7201) -> (-78.4579, -2.7479) construction
  line L300 (-78.4579, -2.7479) -> (-78.4592, -2.7824) construction
  line L301 (-78.4592, -2.7824) -> (-78.4618, -2.8502) construction
  line L302 (-78.4618, -2.8502) -> (-78.4832, -2.9495) construction
  line L303 (-78.4832, -2.9495) -> (-78.5167, -3.0444) construction
  line L304 (-78.5167, -3.0444) -> (-78.565, -3.1337) construction
  line L305 (-78.565, -3.1337) -> (-78.6255, -3.217) construction
  line L306 (-78.6255, -3.217) -> (-78.6996, -3.2916) construction
  line L307 (-78.6996, -3.2916) -> (-78.7854, -3.3587) construction
  line L308 (-78.7854, -3.3587) -> (-78.8498, -3.3947) construction
  line L309 (-78.8498, -3.3947) -> (-78.8828, -3.4132) construction
  line L310 (-78.8828, -3.4132) -> (-78.8601, -3.4206) construction
  line L311 (-78.8601, -3.4206) -> (-78.8157, -3.4352) construction
  line L312 (-78.8157, -3.4352) -> (-78.7525, -3.464) construction
  line L313 (-78.7525, -3.464) -> (-78.6924, -3.4954) construction
  line L314 (-78.6924, -3.4954) -> (-78.6364, -3.5319) construction
  line L315 (-78.6364, -3.5319) -> (-78.584, -3.572) construction
  line L316 (-78.584, -3.572) -> (-78.5355, -3.6161) construction
  line L317 (-78.5355, -3.6161) -> (-78.4907, -3.664) construction
  line L318 (-78.4907, -3.664) -> (-78.4502, -3.716) construction
  line L319 (-78.4502, -3.716) -> (-78.4142, -3.7714) construction
  line L320 (-78.4142, -3.7714) -> (-78.3819, -3.8287) construction
  line L321 (-78.3819, -3.8287) -> (-78.3554, -3.8889) construction
  line L322 (-78.3554, -3.8889) -> (-78.3329, -3.9513) construction
  line L323 (-78.3329, -3.9513) -> (-78.3157, -4.0164) construction
  line L324 (-78.3157, -4.0164) -> (-78.3037, -4.084) construction
  line L325 (-78.3037, -4.084) -> (-78.2967, -4.154) construction
  line L326 (-78.2967, -4.154) -> (-78.2956, -4.2014) construction
  line L327 (-78.2956, -4.2014) -> (-78.2951, -4.2254) construction
  line L328 (-78.2951, -4.2254) -> (-78.2962, -4.2606) construction
  line L329 (-78.2962, -4.2606) -> (-78.2983, -4.3301) construction
  line L330 (-78.2983, -4.3301) -> (-78.312, -4.4324) construction
  line L331 (-78.312, -4.4324) -> (-78.3374, -4.5299) construction
  line L332 (-78.3374, -4.5299) -> (-78.3709, -4.6238) construction
  line L333 (-78.3709, -4.6238) -> (-78.4155, -4.7129) construction
  line L334 (-78.4155, -4.7129) -> (-78.4681, -4.7991) construction
  line L335 (-78.4681, -4.7991) -> (-78.5326, -4.8796) construction
  line L336 (-78.5326, -4.8796) -> (-78.6044, -4.9563) construction
  line L337 (-78.6044, -4.9563) -> (-78.6841, -5.0261) construction
  line L338 (-78.6841, -5.0261) -> (-78.7705, -5.0866) construction
  line L339 (-78.7705, -5.0866) -> (-78.8617, -5.1385) construction
  line L340 (-78.8617, -5.1385) -> (-78.9583, -5.1806) construction
  line L341 (-78.9583, -5.1806) -> (-79.0602, -5.2131) construction
  line L342 (-79.0602, -5.2131) -> (-79.1673, -5.2366) construction
  line L343 (-79.1673, -5.2366) -> (-79.2799, -5.2509) construction
  line L344 (-79.2799, -5.2509) -> (-79.3568, -5.2524) construction
  line L345 (-79.3568, -5.2524) -> (-79.396, -5.2532) construction
  line L346 (-43.5084, -3.1264) -> (-43.4915, -3.1216) construction
  line L347 (-43.4915, -3.1216) -> (-43.4582, -3.1124) construction
  line L348 (-43.4582, -3.1124) -> (-43.408, -3.1031) construction
  line L349 (-43.408, -3.1031) -> (-43.3593, -3.097) construction
  line L350 (-43.3593, -3.097) -> (-43.3274, -3.0962) construction
  line L351 (-43.3274, -3.0962) -> (-43.3119, -3.0958) construction
  line L352 (-43.3119, -3.0958) -> (-43.2781, -3.0966) construction
  line L353 (-43.2781, -3.0966) -> (-43.2116, -3.0981) construction
  line L354 (-43.2116, -3.0981) -> (-43.1142, -3.1126) construction
  line L355 (-43.1142, -3.1126) -> (-43.021, -3.1354) construction
  line L356 (-43.021, -3.1354) -> (-42.9322, -3.1679) construction
  line L357 (-42.9322, -3.1679) -> (-42.8479, -3.2102) construction
  line L358 (-42.8479, -3.2102) -> (-42.768, -3.2614) construction
  line L359 (-42.768, -3.2614) -> (-42.6924, -3.3216) construction
  line L360 (-42.6924, -3.3216) -> (-42.6224, -3.3908) construction
  line L361 (-42.6224, -3.3908) -> (-42.5582, -3.4667) construction
  line L362 (-42.5582, -3.4667) -> (-42.5023, -3.5489) construction
  line L363 (-42.5023, -3.5489) -> (-42.4546, -3.636) construction
  line L364 (-42.4546, -3.636) -> (-42.4166, -3.7288) construction
  line L365 (-42.4166, -3.7288) -> (-42.3866, -3.8265) construction
  line L366 (-42.3866, -3.8265) -> (-42.365, -3.9293) construction
  line L367 (-42.365, -3.9293) -> (-42.3522, -4.0372) construction
  line L368 (-42.3522, -4.0372) -> (-42.3505, -4.1109) construction
  line L369 (-42.3505, -4.1109) -> (-42.3496, -4.1484) construction
  line L370 (-42.3496, -4.1484) -> (-42.3507, -4.1864) construction
  line L371 (-42.3507, -4.1864) -> (-42.3528, -4.2614) construction
  line L372 (-42.3528, -4.2614) -> (-42.3666, -4.3716) construction
  line L373 (-42.3666, -4.3716) -> (-42.3911, -4.4771) construction
  line L374 (-42.3911, -4.4771) -> (-42.4247, -4.5783) construction
  line L375 (-42.4247, -4.5783) -> (-42.4689, -4.6744) construction
  line L376 (-42.4689, -4.6744) -> (-42.5221, -4.7664) construction
  line L377 (-42.5221, -4.7664) -> (-42.5852, -4.8535) construction
  line L378 (-42.5852, -4.8535) -> (-42.6575, -4.935) construction
  line L379 (-42.6575, -4.935) -> (-42.7361, -5.0094) construction
  line L380 (-42.7361, -5.0094) -> (-42.8199, -5.0749) construction
  line L381 (-42.8199, -5.0749) -> (-42.9081, -5.13) construction
  line L382 (-42.9081, -5.13) -> (-43.0008, -5.1746) construction
  line L383 (-43.0008, -5.1746) -> (-43.0975, -5.2098) construction
  line L384 (-43.0975, -5.2098) -> (-43.1982, -5.2355) construction
  line L385 (-43.1982, -5.2355) -> (-43.3034, -5.2502) construction
  line L386 (-43.3034, -5.2502) -> (-43.3748, -5.2522) construction
  line L387 (-43.3748, -5.2522) -> (-43.4111, -5.2532) construction
  line L388 (-43.4111, -5.2532) -> (-43.4436, -5.2524) construction
  line L389 (-43.4436, -5.2524) -> (-43.5076, -5.2507) construction
  line L390 (-43.5076, -5.2507) -> (-43.6019, -5.2407) construction
  line L391 (-43.6019, -5.2407) -> (-43.6928, -5.2229) construction
  line L392 (-43.6928, -5.2229) -> (-43.7798, -5.1972) construction
  line L393 (-43.7798, -5.1972) -> (-43.8639, -5.1655) construction
  line L394 (-43.8639, -5.1655) -> (-43.9441, -5.1259) construction
  line L395 (-43.9441, -5.1259) -> (-44.0208, -5.0791) construction
  line L396 (-44.0208, -5.0791) -> (-44.0938, -5.0259) construction
  line L397 (-44.0938, -5.0259) -> (-44.1619, -4.9661) construction
  line L398 (-44.1619, -4.9661) -> (-44.224, -4.9006) construction
  line L399 (-44.224, -4.9006) -> (-44.2806, -4.8302) construction
  line L400 (-44.2806, -4.8302) -> (-44.3304, -4.7542) construction
  line L401 (-44.3304, -4.7542) -> (-44.3733, -4.6725) construction
  line L402 (-44.3733, -4.6725) -> (-44.4113, -4.5862) construction
  line L403 (-44.4113, -4.5862) -> (-44.4424, -4.4944) construction
  line L404 (-44.4424, -4.4944) -> (-44.4582, -4.4307) construction
  line L405 (-44.4582, -4.4307) -> (-44.4663, -4.3984) construction
  line L406 (-43.815, -4.3984) -> (-43.8031, -4.4208) construction
  line L407 (-43.8031, -4.4208) -> (-43.7799, -4.4644) construction
  line L408 (-43.7799, -4.4644) -> (-43.7359, -4.5222) construction
  line L409 (-43.7359, -4.5222) -> (-43.6866, -4.5715) construction
  line L410 (-43.6866, -4.5715) -> (-43.6326, -4.6128) construction
  line L411 (-43.6326, -4.6128) -> (-43.5733, -4.6438) construction
  line L412 (-43.5733, -4.6438) -> (-43.5113, -4.6672) construction
  line L413 (-43.5113, -4.6672) -> (-43.4458, -4.6808) construction
  line L414 (-43.4458, -4.6808) -> (-43.4012, -4.6825) construction
  line L415 (-43.4012, -4.6825) -> (-43.3787, -4.6833) construction
  line L416 (-43.3787, -4.6833) -> (-43.363, -4.6827) construction
  line L417 (-43.363, -4.6827) -> (-43.3321, -4.6816) construction
  line L418 (-43.3321, -4.6816) -> (-43.2865, -4.6754) construction
  line L419 (-43.2865, -4.6754) -> (-43.2431, -4.6638) construction
  line L420 (-43.2431, -4.6638) -> (-43.2014, -4.6476) construction
  line L421 (-43.2014, -4.6476) -> (-43.1613, -4.6275) construction
  line L422 (-43.1613, -4.6275) -> (-43.1234, -4.6021) construction
  line L423 (-43.1234, -4.6021) -> (-43.0871, -4.5729) construction
  line L424 (-43.0871, -4.5729) -> (-43.0529, -4.5394) construction
  line L425 (-43.0529, -4.5394) -> (-43.0219, -4.502) construction
  line L426 (-43.0219, -4.502) -> (-42.9947, -4.4618) construction
  line L427 (-42.9947, -4.4618) -> (-42.9704, -4.4197) construction
  line L428 (-42.9704, -4.4197) -> (-42.9524, -4.3741) construction
  line L429 (-42.9524, -4.3741) -> (-42.9377, -4.3262) construction
  line L430 (-42.9377, -4.3262) -> (-42.9268, -4.2758) construction
  line L431 (-42.9268, -4.2758) -> (-42.9204, -4.2228) construction
  line L432 (-42.9204, -4.2228) -> (-42.9198, -4.1866) construction
  line L433 (-42.9198, -4.1866) -> (-42.9195, -4.1681) construction
  line L434 (-42.9195, -4.1681) -> (-42.9198, -4.1501) construction
  line L435 (-42.9198, -4.1501) -> (-42.9205, -4.115) construction
  line L436 (-42.9205, -4.115) -> (-42.9262, -4.0635) construction
  line L437 (-42.9262, -4.0635) -> (-42.9365, -4.0146) construction
  line L438 (-42.9365, -4.0146) -> (-42.9504, -3.9679) construction
  line L439 (-42.9504, -3.9679) -> (-42.9683, -3.9238) construction
  line L440 (-42.9683, -3.9238) -> (-42.9901, -3.882) construction
  line L441 (-42.9901, -3.882) -> (-43.016, -3.8427) construction
  line L442 (-43.016, -3.8427) -> (-43.0461, -3.8067) construction
  line L443 (-43.0461, -3.8067) -> (-43.0782, -3.7736) construction
  line L444 (-43.0782, -3.7736) -> (-43.1126, -3.7447) construction
  line L445 (-43.1126, -3.7447) -> (-43.1492, -3.7207) construction
  line L446 (-43.1492, -3.7207) -> (-43.1867, -3.6998) construction
  line L447 (-43.1867, -3.6998) -> (-43.2266, -3.6846) construction
  line L448 (-43.2266, -3.6846) -> (-43.268, -3.6741) construction
  line L449 (-43.268, -3.6741) -> (-43.311, -3.6664) construction
  line L450 (-43.311, -3.6664) -> (-43.3403, -3.6659) construction
  line L451 (-43.3403, -3.6659) -> (-43.3551, -3.6657) construction
  line L452 (-43.3551, -3.6657) -> (-43.3713, -3.6663) construction
  line L453 (-43.3713, -3.6663) -> (-43.4037, -3.6675) construction
  line L454 (-43.4037, -3.6675) -> (-43.4518, -3.6775) construction
  line L455 (-43.4518, -3.6775) -> (-43.4993, -3.6937) construction
  line L456 (-43.4993, -3.6937) -> (-43.5465, -3.716) construction
  line L457 (-43.5465, -3.716) -> (-43.593, -3.7453) construction
  line L458 (-43.593, -3.7453) -> (-43.6399, -3.7795) construction
  line L459 (-43.6399, -3.7795) -> (-43.6856, -3.8213) construction
  line L460 (-43.6856, -3.8213) -> (-43.7147, -3.8525) construction
  line L461 (-43.7147, -3.8525) -> (-43.7297, -3.8686) construction
  line L462 (-25.209, -3.2586) -> (-25.1763, -3.2595) construction
  line L463 (-25.1763, -3.2595) -> (-25.112, -3.2612) construction
  line L464 (-25.112, -3.2612) -> (-25.0172, -3.2746) construction
  line L465 (-25.0172, -3.2746) -> (-24.9266, -3.2979) construction
  line L466 (-24.9266, -3.2979) -> (-24.8393, -3.3288) construction
  line L467 (-24.8393, -3.3288) -> (-24.7563, -3.3703) construction
  line L468 (-24.7563, -3.3703) -> (-24.6763, -3.4196) construction
  line L469 (-24.6763, -3.4196) -> (-24.6014, -3.4797) construction
  line L470 (-24.6014, -3.4797) -> (-24.5297, -3.5464) construction
  line L471 (-24.5297, -3.5464) -> (-24.4646, -3.6202) construction
  line L472 (-24.4646, -3.6202) -> (-24.408, -3.6996) construction
  line L473 (-24.408, -3.6996) -> (-24.3587, -3.7825) construction
  line L474 (-24.3587, -3.7825) -> (-24.3204, -3.8708) construction
  line L475 (-24.3204, -3.8708) -> (-24.2895, -3.9631) construction
  line L476 (-24.2895, -3.9631) -> (-24.2672, -4.0598) construction
  line L477 (-24.2672, -4.0598) -> (-24.2545, -4.161) construction
  line L478 (-24.2545, -4.161) -> (-24.2527, -4.2298) construction
  line L479 (-24.2527, -4.2298) -> (-24.2518, -4.2648) construction
  line L480 (-24.2518, -4.2648) -> (-24.2527, -4.2986) construction
  line L481 (-24.2527, -4.2986) -> (-24.2543, -4.3653) construction
  line L482 (-24.2543, -4.3653) -> (-24.268, -4.4633) construction
  line L483 (-24.268, -4.4633) -> (-24.2901, -4.5573) construction
  line L484 (-24.2901, -4.5573) -> (-24.3217, -4.6471) construction
  line L485 (-24.3217, -4.6471) -> (-24.3618, -4.7333) construction
  line L486 (-24.3618, -4.7333) -> (-24.4109, -4.8156) construction
  line L487 (-24.4109, -4.8156) -> (-24.4694, -4.8936) construction
  line L488 (-24.4694, -4.8936) -> (-24.5357, -4.9668) construction
  line L489 (-24.5357, -4.9668) -> (-24.6082, -5.0335) construction
  line L490 (-24.6082, -5.0335) -> (-24.6846, -5.0927) construction
  line L491 (-24.6846, -5.0927) -> (-24.7655, -5.1417) construction
  line L492 (-24.7655, -5.1417) -> (-24.8495, -5.1831) construction
  line L493 (-24.8495, -5.1831) -> (-24.9381, -5.2139) construction
  line L494 (-24.9381, -5.2139) -> (-25.03, -5.2372) construction
  line L495 (-25.03, -5.2372) -> (-25.1257, -5.2506) construction
  line L496 (-25.1257, -5.2506) -> (-25.1908, -5.2523) construction
  line L497 (-25.1908, -5.2523) -> (-25.2237, -5.2532) construction
  line L498 (-25.2237, -5.2532) -> (-25.2581, -5.2525) construction
  line L499 (-25.2581, -5.2525) -> (-25.3257, -5.2511) construction
  line L500 (-25.3257, -5.2511) -> (-25.4247, -5.2357) construction
  line L501 (-25.4247, -5.2357) -> (-25.5197, -5.2124) construction
  line L502 (-25.5197, -5.2124) -> (-25.61, -5.1792) construction
  line L503 (-25.61, -5.1792) -> (-25.6964, -5.1369) construction
  line L504 (-25.6964, -5.1369) -> (-25.7776, -5.0845) construction
  line L505 (-25.7776, -5.0845) -> (-25.8546, -5.0227) construction
  line L506 (-25.8546, -5.0227) -> (-25.9264, -4.9529) construction
  line L507 (-25.9264, -4.9529) -> (-25.991, -4.8763) construction
  line L508 (-25.991, -4.8763) -> (-26.0487, -4.7969) construction
  line L509 (-26.0487, -4.7969) -> (-26.0975, -4.7143) construction
  line L510 (-26.0975, -4.7143) -> (-26.137, -4.6289) construction
  line L511 (-26.137, -4.6289) -> (-26.1678, -4.5407) construction
  line L512 (-26.1678, -4.5407) -> (-26.1892, -4.4496) construction
  line L513 (-26.1892, -4.4496) -> (-26.2032, -4.356) construction
  line L514 (-26.2032, -4.356) -> (-26.2048, -4.2924) construction
  line L515 (-26.2048, -4.2924) -> (-26.2057, -4.2604) construction
  line L516 (-26.2057, -4.2604) -> (-26.2052, -4.2355) construction
  line L517 (-26.2052, -4.2355) -> (-26.2044, -4.1857) construction
  line L518 (-26.2044, -4.1857) -> (-26.1956, -4.1112) construction
  line L519 (-26.1956, -4.1112) -> (-26.1822, -4.0364) construction
  line L520 (-26.1822, -4.0364) -> (-26.1667, -3.9733) construction
  line L521 (-26.1667, -3.9733) -> (-26.1507, -3.92) construction
  line L522 (-26.1507, -3.92) -> (-26.1346, -3.8748) construction
  line L523 (-26.1346, -3.8748) -> (-26.1147, -3.8247) construction
  line L524 (-26.1147, -3.8247) -> (-26.092, -3.7695) construction
  line L525 (-26.092, -3.7695) -> (-26.0656, -3.7093) construction
  line L526 (-26.0656, -3.7093) -> (-26.0359, -3.6443) construction